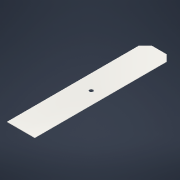
# Autodesk Inventor part: Horquilla_Base
Saved by Autodesk Inventor 2022 (Build 260153000, 153)
## iProperties
Created: 2021-09-10
Part Number: Horquilla_Base
Material: Genérico
Document SubType Name: Modeling
Designer: seb_0
Density: 1 g/cm^3
Appearance: Acero
Author: seb_0
Autodesk Inventor part; units mm, degrees
ref_plane "YZ Plane" through (0, 0, 0) normal (1, 0, 0) x (0, 1, 0)
ref_plane "XZ Plane" through (0, 0, 0) normal (0, 1, 0) x (-1, 0, 0)
ref_plane "XY Plane" through (0, 0, 0) normal (0, 0, 1) x (1, 0, 0)
sketch "Boceto1" plane through (0, 0, 0) normal (0, 1, 0) x (-1, 0, 0)
  line L0 (0, 0) -> (230, 0)
  line L1 (230, 0) -> (230, -1050)
  line L2 (180, -1100) -> (50, -1100)
  line L3 (0, -1050) -> (0, 0)
  line L4 (230, -1050) -> (180, -1100)
  line L5 (0, -1050) -> (50, -1100)
  circle A0 centre (100, -550) radius 15
  circle A1 centre (100, -825) radius 15
  circle A2 centre (100, -275) radius 15
  point P0 (230, -1100)
  point P1 (0, -1100)
  point P2 (115, 0)
  dimension "d0" = 1100
  dimension "d1" = 230
  dimension "d2" = 50
  dimension "d3" = 50
  dimension "d4" = 50
  dimension "d5" = 50
  dimension "d6" = 30
  dimension "d7" = 100
  dimension "d12" = 30
  dimension "d13" = 30
  dimension "d14" = 100
  dimension "d15" = 275
  dimension "d16" = 275
  dimension "d17" = 275
  dimension "d18" = 100
  constraints: 12 end point, 4 point on line, 3 centre point, 2 parallel, 1 horizontal, 1 midpoint, 1 perpendicular
  measures "d0" distance of L0.end point (230, -1100)
  measures "d1" distance of point (230, -1100) point (0, -1100)
  measures "d2" distance of L1.end point (230, -1100)
  measures "d3" distance of L2.start point (230, -1100)
  measures "d4" distance of L3.start point (0, -1100)
  measures "d5" distance of L2.end point (0, -1100)
  measures "d6" diameter of A0
  measures "d7" distance from line of L3 A0.centre
  measures "d12" diameter of A1
  measures "d13" diameter of A2
  measures "d14" distance from line of L3 A2.centre
  measures "d15" distance from line of L0 A2.centre
  measures "d16" distance of A0.centre A2.centre
  measures "d17" distance of A1.centre A0.centre
  measures "d18" distance from line of L3 A1.centre
extrude "Extrusión1" add sketch "Boceto1" along normal blind 1 contours L0 L1 L4 L2 L5 L3 | A1 | A2
sketch "Sketch2" plane through (0, 1, 0) normal (0, 1, 0) x (1, 0, 0)
  line L0 (-50, 1100) -> (-180, 1100) projected
  line L1 (-180, 1100) -> (-230, 1050) projected
  line L2 (-230, 1050) -> (-230, 0) projected
  line L3 (-230, 0) -> (0, 0) projected
  line L4 (0, 0) -> (0, 1050) projected
  line L5 (0, 1050) -> (-50, 1100) projected
  line L6 (-54.1421, 1090) -> (-175.8579, 1090)
  line L7 (-175.8579, 1090) -> (-220, 1045.8579)
  line L8 (-220, 1045.8579) -> (-220, 10)
  line L9 (-220, 10) -> (-10, 10)
  line L10 (-10, 10) -> (-10, 1045.8579)
  line L11 (-10, 1045.8579) -> (-54.1421, 1090)
  line L12 (0, 0) -> (0, 1050) projected
  line L13 (0, 1050) -> (-14.1421, 1050)
  line L14 (-177.9289, 1095) -> (-52.0711, 1095)
  line L15 (-52.0711, 1095) -> (-5, 1047.9289)
  line L16 (-5, 1047.9289) -> (-5, 5)
  line L17 (-5, 5) -> (-225, 5)
  line L18 (-225, 5) -> (-225, 1047.9289)
  line L19 (-225, 1047.9289) -> (-177.9289, 1095)
  dimension "d19" = 10
  dimension "d20" = 5
  constraints: 26 end point, 1 horizontal, 1 point on line, 10 other
  measures "d19" distance between parallel lines of L5 L11
  measures "d20" distance between parallel lines of L6 L14
extrude "Extrusion2" add sketch "Sketch2" along normal blind 50 contours L14 L15 L16 L17 L18 L19
equation "\"d3\" = d2"
equation "\"d4\" = d2"
equation "\"d5\" = d4"
